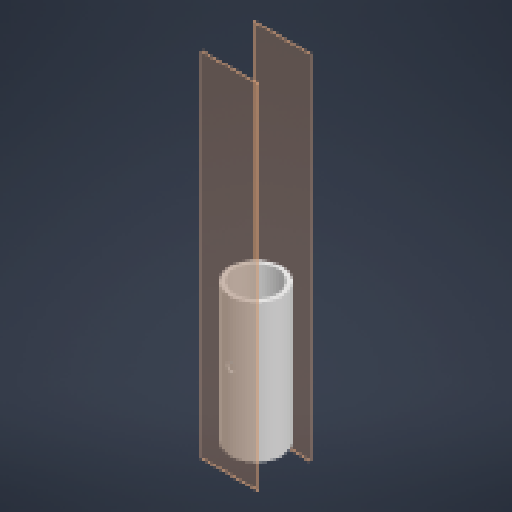
# Autodesk Inventor part: Part4
Saved by Autodesk Inventor 2026.2 (Build 302298000, 298)
## iProperties
Created: 2026-03-11
Part Number: Part4
Material: Generic
Document SubType Name: Modeling
Designer: Alvin
Density: 1 g/cm^3
Appearance: Default
Mass: 24.1855 g
Surface Area: 228.551 cm^2
Volume: 24.1855 cm^3
Author: Alvin
Autodesk Inventor part; units mm, degrees
ref_plane "YZ Plane" through (0, 0, 0) normal (1, 0, 0) x (0, 1, 0)
ref_plane "XZ Plane" through (0, 0, 0) normal (0, 1, 0) x (-1, 0, 0)
sketch "Sketch1" plane through (0, 0, 0) normal (0, 1, 0) x (-1, 0, 0)
  circle A0 centre (0, 0) radius 12.6
  circle A1 centre (0, 0) radius 10.45
  dimension "d0" = 25.2
  dimension "d1" = 20.9
  constraints: 2 centre point, 2 coincident
  measures "d0" diameter of A0
  measures "d1" diameter of A1
extrude "Extrusion1" add sketch "Sketch1" along normal blind 155.5
ref_plane "Work Plane1" through (0, 0, 12.6) normal (0, 0, 1) x (1, 0, 0)
ref_plane "Work Plane2" through (0, 0, -12.6) normal (0, 0, 1) x (1, 0, 0)
sketch "Sketch3" plane through (0, 0, -12.6) normal (0, 0, 1) x (1, 0, 0)
  spline S0 degree 3 poles (-2.2952, 37.46) (-2.2952, 37.7116) (-2.2451, 37.9796) (-2.0416, 38.4723) (-1.8883, 38.6969) (-1.5346, 39.0516) (-1.3105, 39.2054) (-0.8187, 39.4096) (-0.5509, 39.46) (-0.0479, 39.46) (0.2202, 39.4096) (0.7134, 39.2054) (0.9385, 39.0516) (1.294, 38.6969) (1.4483, 38.4723) (1.6531, 37.9796) (1.7037, 37.7116) (1.7037, 37.2084) (1.6531, 36.9404) (1.4483, 36.4477) (1.294, 36.2231) (0.9385, 35.8684) (0.7134, 35.7146) (0.2202, 35.5104) (-0.0479, 35.46) (-0.5509, 35.46) (-0.8187, 35.5104) (-1.3105, 35.7146) (-1.5346, 35.8684) (-1.8883, 36.2231) (-2.0416, 36.4477) (-2.2451, 36.9404) (-2.2952, 37.2084) (-2.2952, 37.46) knots 0 0 0 0 0.07547 0.07547 0.15094 0.15094 0.226409 0.226409 0.301877 0.301877 0.377346 0.377346 0.452814 0.452814 0.528284 0.528284 0.603754 0.603754 0.679224 0.679224 0.754694 0.754694 0.830163 0.830163 0.905632 0.905632 0.9811 0.9811 1.056569 1.056569 1.132039 1.132039 1.207509 1.207509 1.207509 1.207509 projected
  circle A0 centre (0, 37.46) radius 2
  point P0 (0, 0)
  point P1 (-2.2952, 37.46)
  dimension "d6" = 4
  constraints: 1 centre point
  measures "d6" diameter of A0
extrude "Extrusion3" cut sketch "Sketch3" along normal blind 1 contours A0 S0 | S0 A0 picked at (1.8828, 37.6234) picked at (-0.7566, 37.1719)
sketch "Sketch4" plane through (0, 0, 12.6) normal (0, 0, 1) x (1, 0, 0)
  spline S0 degree 3 poles (-1.7037, 37.46) (-1.7037, 37.2084) (-1.6531, 36.9404) (-1.4483, 36.4477) (-1.294, 36.2231) (-0.9385, 35.8684) (-0.7134, 35.7146) (-0.2202, 35.5104) (0.0479, 35.46) (0.5509, 35.46) (0.8187, 35.5104) (1.3105, 35.7146) (1.5346, 35.8684) (1.8883, 36.2231) (2.0416, 36.4477) (2.2451, 36.9404) (2.2952, 37.2084) (2.2952, 37.7116) (2.2451, 37.9796) (2.0416, 38.4723) (1.8883, 38.6969) (1.5346, 39.0516) (1.3105, 39.2054) (0.8187, 39.4096) (0.5509, 39.46) (0.0479, 39.46) (-0.2202, 39.4096) (-0.7134, 39.2054) (-0.9385, 39.0516) (-1.294, 38.6969) (-1.4483, 38.4723) (-1.6531, 37.9796) (-1.7037, 37.7116) (-1.7037, 37.46) knots 0 0 0 0 0.07547 0.07547 0.15094 0.15094 0.226409 0.226409 0.301877 0.301877 0.377346 0.377346 0.452814 0.452814 0.528284 0.528284 0.603754 0.603754 0.679224 0.679224 0.754694 0.754694 0.830163 0.830163 0.905632 0.905632 0.9811 0.9811 1.056569 1.056569 1.132039 1.132039 1.207509 1.207509 1.207509 1.207509 projected
  circle A0 centre (0, 37.46) radius 2
  point P0 (0, 0)
  point P1 (-1.7037, 37.46)
  dimension "d9" = 4
  constraints: 1 centre point
  measures "d9" diameter of A0
extrude "Extrusion4" cut sketch "Sketch4" against normal blind 1 contours S0 A0 | S0 A0 picked at (-0.4487, 37.2971) picked at (-1.7637, 37.1417)
move faces "Move1" translate (0, -12.5, 0) faces at (-11.6601, 155.5, -1.8387)
move faces "Move2" translate (0, -75.8, 0) faces at (-11.7613, 143, 1.0051)
move faces "Move3" translate (0, 75.8, 0) faces at (-11.7613, 67.2, 1.0051)
move faces "Move4" translate (0, -75.8, 0) faces at (-11.7613, 143, 1.0051)
sketch "Sketch5" plane through (0, 0, 0) normal (0, -1, 0) x (1, 0, 0)
  point P0 (0, 0)
sketch "Sketch6" plane through (0, 37.46, -11.6) normal (0, 0, -1) x (-1, 0, 0)
  circle A0 centre (0, 0) radius 2 projected
  point P0 (0, -37.46)
extrude "Extrusion5" add sketch "Sketch6" along normal up to surface round surface about axis through (0, 0, 0) along (0, 1, 0) radius 12.6 far side no
sketch "Sketch7" plane through (0, 37.46, 11.6) normal (0, 0, 1) x (1, 0, 0)
  circle A0 centre (0, 0) radius 2 projected
  point P0 (0, -37.46)
extrude "Extrusion6" add sketch "Sketch7" along normal up to surface round surface about axis through (0, 0, 0) along (0, 1, 0) radius 12.6 far side no
body "Solid1"
